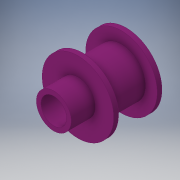
# Autodesk Inventor part: IdlePully
Saved by Autodesk Inventor 2019 (Build 230136000, 136)
## iProperties
Created: 2019-10-03
Part Number: IdlePully
Material: Generic
Document SubType Name: Modeling
Designer: james
Density: 1 g/cm^3
Appearance: Default(1)
Author: james
Autodesk Inventor part; units mm, degrees
ref_plane "YZ Plane" through (0, 0, 0) normal (1, 0, 0) x (0, 1, 0)
ref_plane "XZ Plane" through (0, 0, 0) normal (0, 1, 0) x (-1, 0, 0)
ref_plane "XY Plane" through (0, 0, 0) normal (0, 0, 1) x (1, 0, 0)
sketch "Sketch1" plane through (0, 0, 0) normal (1, 0, 0) x (0, 1, 0)
  line L0 (18.9706, -3.0956) -> (18.9706, 15.9544)
  line L1 (18.9706, 15.9544) -> (23.5426, 15.9544)
  line L2 (23.5426, 15.9544) -> (23.5426, 9.6044)
  line L3 (23.5426, 9.6044) -> (28.3686, 9.6044)
  line L4 (28.3686, 9.6044) -> (28.3686, 8.3344)
  line L5 (28.3686, 8.3344) -> (25.3206, 8.3344)
  line L6 (25.3206, 8.3344) -> (25.3206, -1.8256)
  line L7 (25.3206, -1.8256) -> (28.3686, -1.8256)
  line L8 (28.3686, -1.8256) -> (28.3686, -3.0956)
  line L9 (28.3686, -3.0956) -> (18.9706, -3.0956)
  point P0 (0, 0)
  dimension "d0" = 1.27
  dimension "d1" = 1.27
  dimension "d2" = 10.16
  dimension "d3" = 6.35
  dimension "d6" = 9.398
  dimension "d11" = 6.35
  dimension "d12" = 4.572
  constraints: 20 end point, 8 perpendicular, 2 point on line, 1 vertical
  measures "d0" distance between parallel lines of L3 L5
  measures "d1" distance between parallel lines of L9 L7
  measures "d2" distance of L5.end L6.end
  measures "d3" distance of L1.end L2.end
  measures "d6" distance between parallel lines of L0 L4
  measures "d11" distance between parallel lines of L0 L6
  measures "d12" distance between parallel lines of L0 L2
revolve "Revolution1" add sketch "Sketch1" angle 360 about axis through (0, 18.9706, -3.0956) along (0, 0, 1)
sketch "Sketch2" plane through (0, 18.9706, -3.0956) normal (0, 0, -1) x (-1, 0, 0)
  circle A0 centre (0, 0) radius 9.398 projected
  circle A1 centre (0, 0) radius 3.3909
  point P0 (0, -18.9706)
  dimension "d8" = 6.7818
  constraints: 1 centre point, 1 coincident
  measures "d8" diameter of A1
extrude "Extrusion1" cut sketch "Sketch2" against normal blind 50.8 contours A1
body "Solid1"
